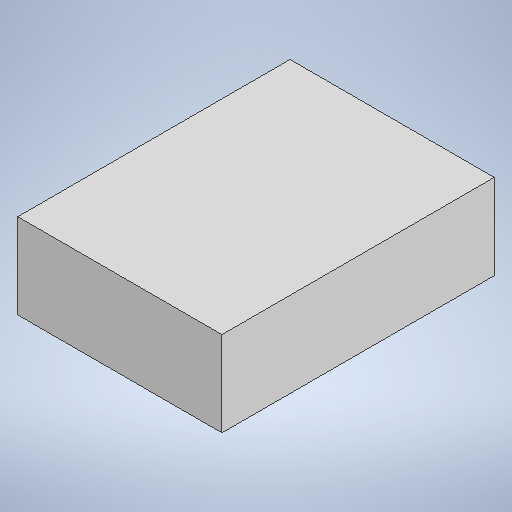
# Autodesk Inventor part: ControlPanel
Saved by Autodesk Inventor 2025.1 (Build 291241000, 241)
## iProperties
Created: 2025-02-25
Part Number: ControlPanel
Material: Generic
Document SubType Name: Modeling
Designer: yovan
Density: 1 g/cm^3
Appearance: Default
Author: yovan
Autodesk Inventor part; units mm, degrees
ref_plane "YZ Plane" through (0, 0, 0) normal (1, 0, 0) x (0, 1, 0)
ref_plane "XZ Plane" through (0, 0, 0) normal (0, 1, 0) x (-1, 0, 0)
ref_plane "XY Plane" through (0, 0, 0) normal (0, 0, 1) x (1, 0, 0)
sketch "Sketch1" plane through (0, 0, 0) normal (0, 0, 1) x (1, 0, 0)
  line L0 (0, 0) -> (600, 0)
  line L1 (600, 0) -> (600, 250)
  line L2 (600, 250) -> (0, 250)
  line L3 (0, 250) -> (0, 0)
  dimension "d0" = 600
  dimension "d1" = 250
  constraints: 8 end point, 2 parallel, 1 horizontal, 1 perpendicular
  measures "d0" distance of L2.end L1.end
  measures "d1" distance of L1.end L0.end
extrude "Extrusion1" add sketch "Sketch1" along normal blind 800
sketch "Sketch2" plane through (0, 0, 0) normal (0, -1, 0) x (1, 0, 0)
  line L0 (0, 0) -> (600, 0)
  line L1 (600, 0) -> (600, 800)
  line L2 (600, 800) -> (0, 800)
  line L3 (0, 800) -> (0, 0)
  line L4 (90, 710) -> (510, 710)
  line L5 (510, 710) -> (510, 90)
  line L6 (510, 90) -> (90, 90)
  line L7 (90, 90) -> (90, 710)
  line L8 (300, 710) -> (300, 90)
  line L9 (90, 400) -> (510, 400)
  line L10 (90, 710) -> (90, 400)
  line L11 (90, 400) -> (90, 90)
  line L12 (90, 555) -> (510, 555)
  line L13 (90, 245) -> (510, 245)
  line L14 (90, 710) -> (300, 710)
  line L15 (300, 710) -> (300, 555)
  line L16 (300, 555) -> (90, 555)
  line L17 (90, 555) -> (90, 710)
  line L18 (300, 555) -> (510, 555)
  line L19 (510, 555) -> (510, 710)
  line L20 (510, 710) -> (300, 710)
  line L21 (300, 710) -> (300, 555)
  line L22 (90, 555) -> (300, 555)
  line L23 (300, 555) -> (300, 400)
  line L24 (300, 400) -> (90, 400)
  line L25 (90, 400) -> (90, 555)
  line L26 (300, 400) -> (510, 400)
  line L27 (510, 400) -> (510, 555)
  line L28 (510, 555) -> (300, 555)
  line L29 (300, 555) -> (300, 400)
  line L30 (510, 400) -> (300, 400)
  line L31 (300, 400) -> (300, 245)
  line L32 (300, 245) -> (510, 245)
  line L33 (510, 245) -> (510, 400)
  line L34 (90, 400) -> (300, 400)
  line L35 (300, 400) -> (300, 245)
  line L36 (300, 245) -> (90, 245)
  line L37 (90, 245) -> (90, 400)
  line L38 (90, 90) -> (300, 90)
  line L39 (300, 90) -> (300, 245)
  line L40 (300, 245) -> (90, 245)
  line L41 (90, 245) -> (90, 90)
  line L42 (300, 245) -> (510, 245)
  line L43 (510, 245) -> (510, 90)
  line L44 (510, 90) -> (300, 90)
  line L45 (300, 90) -> (300, 245)
  line L46 (90, 632.5) -> (510, 632.5)
  line L47 (90, 477.5) -> (510, 477.5)
  line L48 (90, 322.5) -> (510, 322.5)
  line L49 (90, 167.5) -> (510, 167.5)
  line L50 (195, 710) -> (195, 90)
  line L51 (405, 710) -> (405, 90)
  circle A0 centre (195, 632.5) radius 20
  circle A1 centre (300, 632.5) radius 20
  circle A2 centre (405, 632.5) radius 20
  circle A3 centre (90, 632.5) radius 20
  circle A4 centre (510, 632.5) radius 20
  circle A5 centre (90, 477.5) radius 17.5
  circle A6 centre (195, 477.5) radius 17.5
  circle A7 centre (300, 477.5) radius 17.5
  circle A8 centre (405, 477.5) radius 17.5
  circle A9 centre (510, 477.5) radius 17.5
  circle A10 centre (195, 322.5) radius 20
  dimension "d4" = 90
  dimension "d5" = 40
  dimension "d6" = 40
  dimension "d7" = 40
  dimension "d8" = 40
  dimension "d9" = 40
  dimension "d10" = 35
  dimension "d11" = 35
  dimension "d12" = 35
  dimension "d13" = 35
  dimension "d14" = 35
  dimension "d15" = 40
  constraints: 104 end point, 23 midpoint, 20 parallel, 14 perpendicular, 12 point on line, 11 centre point, 9 horizontal, 4 coincident, 3 other
  measures "d4" distance between parallel lines of L2 L4
  measures "d5" diameter of A0
  measures "d6" diameter of A1
  measures "d7" diameter of A2
  measures "d8" diameter of A3
  measures "d9" diameter of A4
  measures "d10" diameter of A5
  measures "d11" diameter of A6
  measures "d12" diameter of A7
  measures "d13" diameter of A8
  measures "d14" diameter of A9
  measures "d15" diameter of A10
extrude "Extrusion2" add sketch "Sketch2" along normal blind 15 contours A3 L46 L7 | L7 A3 | A0 L46 L50 | L50 L46 A0 | L46 A3 L7 | A1 L46 L8 | L8 L46 A1 | L50 A0 L46 | L46 A0 L50 | A2 L46 L51 | L51 L46 A2 | L46 A1 L8 | L8 A1 L46 | A4 L5 | L5 L46 A4 | L51 A2 L46 | L46 A2 L51 | L5 A4 L46
extrude "Extrusion3" add sketch "Sketch2" along normal blind 10 contours A5 L47 L7 | L7 A5 | L47 A5 L7 | A6 L47 L50 | L50 L47 A6 | L47 L50 A6 | A7 L47 L8 | L8 L47 A7 | L47 A6 L50 | L47 A7 L8 | L8 A7 L47 | A8 L47 L51 | L51 L47 A8 | L47 L51 A8 | A9 L5 | L5 L47 A9 | L47 A8 L51 | L5 A9 L47
extrude "Extrusion4" add sketch "Sketch2" along normal blind 20 contours A10 L50 L48 | L48 L50 A10 | A10 L48 L50 | L48 A10 L50
sketch "Sketch3" plane through (195, -10, 477.5) normal (0, -1, 0) x (1, 0, 0)
  circle A0 centre (-105, 0) radius 17.5 projected
  circle A1 centre (-105, 0) radius 15
  circle A2 centre (0, 0) radius 17.5 projected
  circle A3 centre (0, 0) radius 15
  circle A4 centre (105, 0) radius 17.5 projected
  circle A5 centre (105, 0) radius 15
  circle A6 centre (210, 0) radius 17.5 projected
  circle A7 centre (210, 0) radius 15
  circle A8 centre (315, 0) radius 17.5 projected
  circle A9 centre (315, 0) radius 15
  point P0 (-195, -477.5)
  dimension "d22" = 30
  dimension "d23" = 30
  dimension "d24" = 30
  dimension "d25" = 30
  dimension "d26" = 30
  constraints: 5 centre point, 5 coincident
  measures "d22" diameter of A1
  measures "d23" diameter of A3
  measures "d24" diameter of A5
  measures "d25" diameter of A7
  measures "d26" diameter of A9
extrude "Extrusion5" cut sketch "Sketch3" against normal blind 2 contours A1 | A3 | A5 | A7 | A9
sketch "Sketch4" plane through (195, -20, 322.5) normal (0, -1, 0) x (1, 0, 0)
  circle A0 centre (0, 0) radius 30
  point P0 (-195, -322.5)
  dimension "d29" = 60
  constraints: 1 centre point
  measures "d29" diameter of A0
extrude "Extrusion6" add sketch "Sketch4" along normal blind 30
body "Solid1"
